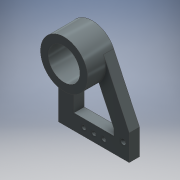
# Autodesk Inventor part: chassi_front_right
Saved by Autodesk Inventor 2016 (Build 200138000, 138)
## iProperties
Created: 2017-01-01
Part Number: chassi_front_right
Material: Generic
Document SubType Name: Modeling
Designer: hesaon
Density: 1 g/cm^3
Appearance: Default
Author: hesaon
Autodesk Inventor part; units mm, degrees
ref_plane "YZ Plane" through (0, 0, 0) normal (1, 0, 0) x (0, 1, 0)
ref_plane "XZ Plane" through (0, 0, 0) normal (0, 1, 0) x (-1, 0, 0)
ref_plane "XY Plane" through (0, 0, 0) normal (0, 0, 1) x (1, 0, 0)
sketch "Sketch1" plane through (0, 0, 0) normal (0, 1, 0) x (-1, 0, 0)
  line L0 (-55, -52.5) -> (-24.8972, 11.6781)
  line L1 (-55, -82.5) -> (-55, -52.5)
  line L2 (27.5, 0) -> (27.5, -82.5)
  line L3 (9.5, -64.5) -> (-37, -64.5)
  line L4 (9.5, -64.5) -> (9.5, -25.807)
  line L5 (-37, -64.5) -> (-37, -56.5118)
  arc A0 (27.5, 0) -> (-24.8972, 11.6781) centre (0, 0) ccw
  arc A1 (-19.56, -19.3302) -> (9.5, -25.807) centre (0, 0) ccw
  circle A2 centre (0, 7) radius 6.25
  circle A3 centre (15.5, 0) radius 1.6
  circle A4 centre (7.75, 13.4234) radius 1.6
  circle A5 centre (-7.75, 13.4234) radius 1.6
  circle A6 centre (-15.5, 0) radius 1.6
  circle A7 centre (-7.75, -13.4234) radius 1.6
  circle A8 centre (7.75, -13.4234) radius 1.6
  line L6 (-19.56, -19.3302) -> (-37, -56.5118)
  line L7 (27.5, -82.5) -> (-55, -82.5)
  dimension "d12" = 18
  dimension "d13" = 82.5
  dimension "d14" = 12.5
  dimension "d15" = 7
  dimension "d16" = 3.2
  dimension "d17" = 15.5
  dimension "d20" = 360
  dimension "d22" = 30
  dimension "d23" = 27.5
  dimension "d24" = 18
  dimension "d25" = 27.5
  dimension "d26" = 27.5
  dimension "d27" = 27.5
  dimension "d29" = 18
  dimension "d30" = 18
  dimension "d31" = 82.5
  dimension "d32" = 82.5
  constraints: 16 end point, 9 centre point, 4 point on circle, 3 vertical, 2 horizontal, 2 tangent, 1 horizontal alignment, 1 parallel, 1 vertical alignment, 13 other
  measures "d12" distance from line of L1 L3.end
  measures "d13" distance of L2.end L1.start
  measures "d14" diameter of A2
  measures "d15" distance of point (0, 0) A2.centre
  measures "d16" diameter of A3
  measures "d17" distance of point (0, 0) A3.centre
  measures "d22" distance of L1.start L0.start
  measures "d23" radius of A0
  measures "d24" distance between parallel lines of L4 L2
  measures "d25" radius of A1
  measures "d26" distance of L2.start point (0, 0)
  measures "d27" distance from line of L0 point (0, 0)
  measures "d29" distance between parallel lines of L0 L6
  measures "d30" distance between parallel lines of L7 L3
  measures "d31" distance from line of point (0, 0) L7
  measures "d32" distance of L2.end L2.start
extrude "Extrusion1" add sketch "Sketch1" along normal blind 6
sketch "Sketch2" plane through (0, 0, 0) normal (0, -1, 0) x (1, 0, 0)
  arc A0 (24.8972, 11.6781) -> (-27.5, 0) centre (0, 0) ccw projected
  circle A1 centre (0, 0) radius 27.5
  circle A2 centre (0, 0) radius 18.5
  dimension "d35" = 37
  constraints: 2 centre point, 2 coincident, 1 concentric
  measures "d35" diameter of A2
extrude "Extrusion2" add sketch "Sketch2" along normal blind 27
sketch "Sketch5" plane through (0, 0, 0) normal (0, -1, 0) x (1, 0, 0)
  line L0 (-27.5, -82.5) -> (-27.5, 0) projected
  line L1 (-27.5, 0) -> (-27.5, -82.5)
  line L2 (55, -82.5) -> (-27.5, -82.5) projected
  line L3 (-27.5, -82.5) -> (55, -82.5)
  line L4 (55, -82.5) -> (55, -52.5)
  line L5 (24.8972, 11.6781) -> (55, -52.5) projected
  line L6 (55, -52.5) -> (24.8972, 11.6781)
  line L7 (37, -56.5118) -> (19.56, -19.3302) projected
  line L8 (19.56, -19.3302) -> (37, -56.5118)
  line L9 (37, -64.5) -> (37, -56.5118) projected
  line L10 (37, -56.5118) -> (37, -64.5)
  line L11 (-9.5, -25.807) -> (-9.5, -64.5) projected
  line L12 (37, -64.5) -> (-9.5, -64.5)
  line L13 (-9.5, -64.5) -> (-9.5, -25.807)
  arc A0 (19.56, -19.3302) -> (24.8972, 11.6781) centre (0, 0) ccw
  arc A1 (-27.5, 0) -> (-9.5, -25.807) centre (0, 0) ccw
  constraints: 16 end point, 4 collinear, 4 point on circle, 3 perpendicular, 2 centre point, 1 coincident, 1 vertical
extrude "Extrusion5" add sketch "Sketch5" along normal blind 6
sketch "Sketch7" plane through (0, -6, 0) normal (0, -1, 0) x (1, 0, 0)
  circle A0 centre (2.125, -73.5) radius 2.5
  circle A1 centre (13.75, -73.5) radius 2.5
  line L0 (-9.5, -64.5) -> (-9.5, -25.807) projected
  line L1 (37, -64.5) -> (-9.5, -64.5) projected
  circle A2 centre (25.375, -73.5) radius 2.5
  line L2 (37, -56.5118) -> (37, -64.5) projected
  point P0 (0, 0)
  dimension "d63" = 5
  dimension "d64" = 5
  dimension "d65" = 11.625
  dimension "d66" = 11.625
  dimension "d67" = 9
  dimension "d73" = 5
  dimension "d85" = 11.625
  constraints: 3 centre point, 2 horizontal alignment
  measures "d63" diameter of A0
  measures "d64" diameter of A1
  measures "d65" distance of A1.centre A0.centre
  measures "d66" distance from line of A0.centre L0
  measures "d67" distance from line of L1 A0.centre
  measures "d73" diameter of A2
  measures "d85" distance of A2.centre A1.centre
extrude "Extrusion8" cut sketch "Sketch7" against normal up to next
sketch "Sketch8" plane through (0, -6, 0) normal (0, -1, 0) x (1, 0, 0)
  circle A0 centre (48, -65) radius 3
  line L0 (55, -82.5) -> (55, -52.5) projected
  line L1 (-27.5, -82.5) -> (55, -82.5) projected
  point P0 (0, 0)
  dimension "d88" = 6
  dimension "d89" = 7
  dimension "d90" = 17.5
  constraints: 1 centre point
  measures "d88" diameter of A0
  measures "d89" distance from line of L0 A0.centre
  measures "d90" distance from line of L1 A0.centre
extrude "Extrusion9" cut sketch "Sketch8" against normal through all
sketch "Sketch10" plane through (0, 6, 0) normal (0, 1, 0) x (1, 0, 0)
  circle A0 centre (48, 65) radius 3 projected
  line L0 (42.8, 61.9978) -> (42.8, 68.0022)
  line L1 (42.8, 68.0022) -> (48, 71.0044)
  line L2 (48, 71.0044) -> (53.2, 68.0022)
  line L3 (53.2, 68.0022) -> (53.2, 61.9978)
  line L4 (53.2, 61.9978) -> (48, 58.9956)
  line L5 (48, 58.9956) -> (42.8, 61.9978)
  line L6 (55, 52.5) -> (55, 82.5) projected
  point P0 (0, 0)
  dimension "d94" = 10.4
  constraints: 12 end point, 1 coincident, 1 parallel, 13 other
  measures "d94" distance between parallel lines of L0 L3
extrude "Extrusion10" cut sketch "Sketch10" against normal blind 5
body "Solid1"
